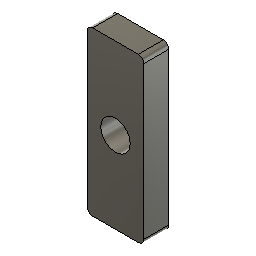
SpeedClip_Configured_v39 (Autodesk Fusion 360 archive; units mm, degrees)
design "Long Nut"
Autodesk Fusion 360 part; units mm, degrees
sketch "Sketch1" plane through (0, 0, 0) normal (0, 0, 1) x (1, 0, 0)
  line L0 (2.6, 7.5) -> (-2.6, 7.5)
  line L1 (-2.6, 7.5) -> (-2.6, -7.5)
  line L2 (-2.6, -7.5) -> (2.6, -7.5)
  line L3 (2.6, -7.5) -> (2.6, 7.5)
  line L4 (2.6, 7.5) -> (-2.6, -7.5) construction
  line L5 (-2.6, 7.5) -> (2.6, -7.5) construction
  circle A0 centre (0, 0) radius 1.35
  dimension "d1" = 5.2
  dimension "d2" = 15
  dimension "d3" = 2.7
  constraint horizontal L0
  constraint perpendicular L0 L1
  constraint parallel L0 L2
  constraint parallel L1 L3
  constraint coincident L4 A0.centre
  constraint coincident L5 A0.centre
  constraint coincident A0.centre origin
  measures "d1" distance of L0.start L0.end
  measures "d2" distance of L0.start L2.end
  measures "d3" diameter of A0
extrude "Extrude1" add sketch "Sketch1" along normal blind 2.3
fillet "Fillet1" radius 0.5 4 edges at (2.6, 7.5, 1.15) (-2.6, 7.5, 1.15) (-2.6, -7.5, 1.15) (2.6, -7.5, 1.15)
